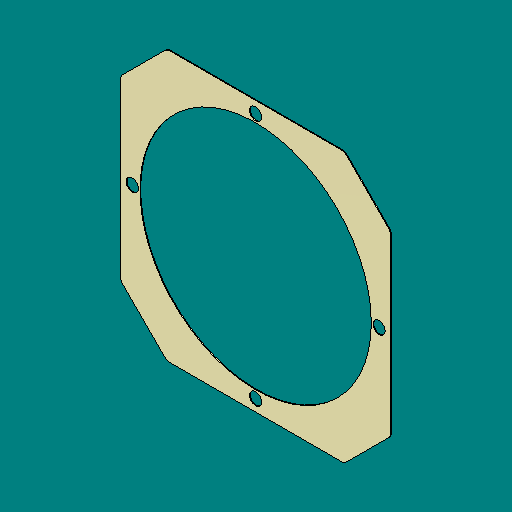
# Autodesk Inventor part: plasma-box-mica
Saved by Autodesk Inventor 2025 (Build 290162000, 162)
## iProperties
Created: 2024-06-26
Part Number: plasma-box-mica
Material: Nylon 6/6
Document SubType Name: Modeling
Designer: kuzmin
Density: 1.13 g/cm^3
Appearance: Nylon 6
Author: kuzmin
Autodesk Inventor part; units mm, degrees
ref_plane "YZ Plane" through (0, 0, 0) normal (1, 0, 0) x (0, 1, 0)
ref_plane "XZ Plane" through (0, 0, 0) normal (0, 1, 0) x (-1, 0, 0)
ref_plane "XY Plane" through (0, 0, 0) normal (0, 0, 1) x (1, 0, 0)
sketch "Sketch1" plane through (0, 0, 0) normal (0, 0, 1) x (1, 0, 0)
  line L0 (-35, 35) -> (35, 35)
  line L1 (35, 35) -> (35, -35)
  line L2 (35, -35) -> (-35, -35)
  line L3 (-35, -35) -> (-35, 35)
  circle A0 centre (0, 0) radius 30
  point P0 (35, 0)
  point P1 (0, 35)
  dimension "d0" = 70
  dimension "d1" = 60
  constraints: 8 end point, 2 midpoint, 2 parallel, 2 perpendicular, 1 centre point, 1 coincident, 1 horizontal, 1 horizontal alignment, 1 vertical alignment
  measures "d0" distance of L0.start L0.end
  measures "d1" diameter of A0
extrude "Extrusion1" add sketch "Sketch1" along normal blind 0.2
chamfer "Chamfer1" distance 12 angle 45 4 edges at (35, 35, 0.1) (35, -35, 0.1) (-35, -35, 0.1) (-35, 35, 0.1)
fillet "Fillet1" radius 2 8 edges at (-23, 35, 0.1) (23, 35, 0.1) (35, 23, 0.1) (35, -23, 0.1) (23, -35, 0.1) (-23, -35, 0.1) (-35, -23, 0.1) (-35, 23, 0.1)
sketch "Sketch2" plane through (0, 0, 0.2) normal (0, 0, 1) x (1, 0, 0)
  circle A0 centre (0, 0) radius 32 construction
  point P0 (32, 0)
  dimension "d8" = 64
  constraints: 2 horizontal alignment, 1 coincident, 2 other
hole "Hole1" at (32, 0, 0.2) direction (0, 0, -1) diameter 3.2 end through all
pattern_circular "Circular Pattern1" count 4 over 360 about axis through (0, 0, -10) along (0, 0, 1) of "Hole1"
sketch "Sketch3" plane through (0, 0, 0.2) normal (0, 0, 1) x (1, 0, 0)
  circle A0 centre (0, 0) radius 23.75 construction
  point P0 (23.75, 0)
  dimension "d19" = 47.5
  constraints: 2 horizontal alignment, 1 coincident, 2 other
body "Solid1"
